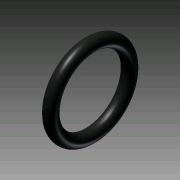
# Autodesk Inventor part: O Ring 2 R.671 1764
Saved by Autodesk Inventor 2011 (Build 150239000, 239)
## iProperties
Created: 2007-11-29
Part Number: O Ring 2 R.671 1764
Document SubType Name: Modeling
Designer: lwoods
Density: 1 g/cm^3
Author: lwoods
Autodesk Inventor part; units mm, degrees
ref_plane "YZ Plane" through (0, 0, 0) normal (1, 0, 0) x (0, 1, 0)
ref_plane "XZ Plane" through (0, 0, 0) normal (0, 1, 0) x (-1, 0, 0)
ref_plane "XY Plane" through (0, 0, 0) normal (0, 0, 1) x (1, 0, 0)
sketch "Sketch1" plane through (0, 0, 0) normal (0, 0, 1) x (1, 0, 0)
  circle A0 centre (-6.4516, 7.037) radius 1.5875
  line L0 (-23.4255, -3.0722) -> (10.3687, -3.0722)
  line L1 (-6.4516, 7.037) -> (-6.4516, 5.4495)
  line L2 (-6.4516, 5.4495) -> (-6.4516, -3.0722)
  dimension "d0" = 3.175
  dimension "d1" = 8.5217
  constraints: 6 end point, 2 perpendicular, 1 horizontal, 1 point on line, 1 vertical alignment, 2 other
  measures "d1" distance of L2.end L1.end
revolve "Revolution1" add sketch "Sketch1" angle 360 about axis through (-23.4255, -3.0722, 0) along (1, 0, 0)
body "Solid1"
